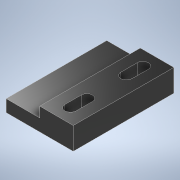
# Autodesk Inventor part: 59145_Actuator
Saved by Autodesk Inventor 2021 (Build 250183000, 183)
## iProperties
Created: 2021-10-07
Part Number: 59145_Actuator
Material: Generic
Document SubType Name: Modeling
Designer: Jorian Brusind
Density: 1 g/cm^3
Appearance: Glossy - Black
Author: Jorian Brusind
Autodesk Inventor part; units mm, degrees
ref_plane "YZ Plane" through (0, 0, 0) normal (1, 0, 0) x (0, 1, 0)
ref_plane "XZ Plane" through (0, 0, 0) normal (0, 1, 0) x (-1, 0, 0)
ref_plane "XY Plane" through (0, 0, 0) normal (0, 0, 1) x (1, 0, 0)
sketch "Sketch1" plane through (0, 0, 0) normal (0, 1, 0) x (-1, 0, 0)
  line L0 (0, 0) -> (19.05, 0)
  line L1 (19.05, 0) -> (19.05, -28.57)
  line L2 (19.05, -28.57) -> (0, -28.57)
  line L3 (0, -28.57) -> (0, 0)
  dimension "d0" = 19.05
  dimension "d1" = 28.57
  constraints: 8 end point, 2 parallel, 1 horizontal, 1 perpendicular
  measures "d0" distance of L1.end L2.end
  measures "d1" distance of L0.end L1.end
extrude "Extrusion1" add sketch "Sketch1" along normal blind 3.43
sketch "Sketch2" plane through (0, 3.43, 0) normal (0, 1, 0) x (1, 0, 0)
  line L0 (0, 28.57) -> (-19.05, 28.57) projected
  line L1 (0, 0) -> (-9.53, 0)
  line L2 (-9.53, 0) -> (-9.53, 28.57)
  line L3 (-9.53, 28.57) -> (0, 28.57)
  line L4 (0, 28.57) -> (0, 0)
  dimension "d4" = 9.53
  constraints: 8 end point, 2 parallel, 1 horizontal, 1 perpendicular, 1 point on line
  measures "d4" distance of L2.end L3.end
extrude "Extrusion2" add sketch "Sketch2" along normal blind 2.92
sketch "Sketch3" plane through (0, 6.35, 0) normal (0, 1, 0) x (1, 0, 0)
  line L0 (-4.77, 4.02) -> (-4.77, 8.66) construction
  line L1 (-3.18, 4.02) -> (-3.18, 8.66)
  line L2 (-6.36, 8.66) -> (-6.36, 4.02)
  arc A0 (-6.36, 4.02) -> (-3.18, 4.02) centre (-4.77, 4.02) ccw
  arc A1 (-3.18, 8.66) -> (-6.36, 8.66) centre (-4.77, 8.66) ccw
  line L3 (-19.05, 28.57) -> (-19.05, 0) projected
  line L4 (-4.77, 19.9) -> (-4.77, 24.54) construction
  line L5 (-3.18, 19.9) -> (-3.18, 24.54)
  line L6 (-6.36, 24.54) -> (-6.36, 19.9)
  arc A2 (-6.36, 19.9) -> (-3.18, 19.9) centre (-4.77, 19.9) ccw
  arc A3 (-3.18, 24.54) -> (-6.36, 24.54) centre (-4.77, 24.54) ccw
  line L7 (0, 28.57) -> (-9.53, 28.57) projected
  point P0 (0, 0)
  point P1 (-4.77, 6.34)
  point P2 (-4.77, 22.22)
  dimension "d7" = 4.64
  dimension "d8" = 3.18
  dimension "d9" = 14.28
  dimension "d10" = 4.64
  dimension "d11" = 3.18
  dimension "d12" = 15.88
  dimension "d13" = 6.35
  constraints: 16 end point, 8 point on circle, 8 tangent, 4 centre point, 2 midpoint, 2 parallel, 2 vertical
  measures "d7" distance of L0.start L0.end
  measures "d8" diameter of A1
  measures "d9" distance from line of L3 point (-4.77, 6.34)
  measures "d10" distance of L4.start L4.end
  measures "d11" diameter of A3
  measures "d12" distance of point (-4.77, 22.22) point (-4.77, 6.34)
  measures "d13" distance from line of L7 point (-4.77, 22.22)
extrude "Extrusion3" cut sketch "Sketch3" against normal through all
body "Solid1"
